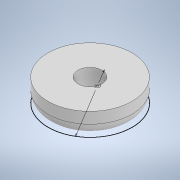
# Autodesk Inventor part: RoundRetainingClip
Saved by Autodesk Inventor 2020 (Build 240168000, 168)
## iProperties
Created: 2023-02-18
Part Number: RoundRetainingClip
Material: Generic
Document SubType Name: Modeling
Designer: Beaucage
Density: 1 g/cm^3
Appearance: Default
Author: Beaucage
Autodesk Inventor part; units mm, degrees
ref_plane "YZ Plane" through (0, 0, 0) normal (1, 0, 0) x (0, 1, 0)
ref_plane "XZ Plane" through (0, 0, 0) normal (0, 1, 0) x (-1, 0, 0)
ref_plane "XY Plane" through (0, 0, 0) normal (0, 0, 1) x (1, 0, 0)
sketch "Sketch1" plane through (0, 0, 0) normal (0, 1, 0) x (-1, 0, 0)
  circle A0 centre (0, 0) radius 11.8999
  dimension "d0" = 23.7998
  constraints: 1 centre point, 1 coincident
  measures "d0" diameter of A0
extrude "Extrusion1" add sketch "Sketch1" along normal blind 6.35
hole "Hole1" at (0, 0, 0) direction (0, 1, 0) diameter 6.7564 end through all counterbore diameter 11.1252 counterbore depth 1.5875 clearance for "Socket Head Cap Screw" size "1/4" standard "Ansi Unified Screw Threads"
fillet "Fillet1" radius 3.175 1 edges at (11.8999, 0, 0)
body "Solid1"
